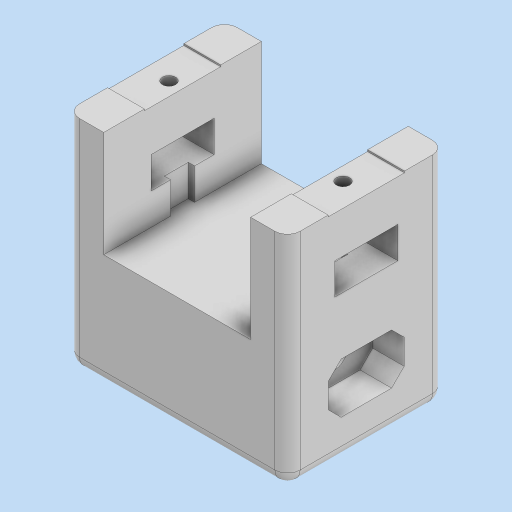
# Autodesk Inventor part: Base_Motor_Hombro2
Saved by Autodesk Inventor 2024 (Build 280153000, 153)
## iProperties
Created: 2024-07-27
Part Number: Base_Motor_Hombro2
Material: Generic
Document SubType Name: Modeling
Designer: MxMon
Density: 1 g/cm^3
Appearance: Default
Author: MxMon
Autodesk Inventor part; units mm, degrees
ref_plane "YZ Plane" through (0, 0, 0) normal (1, 0, 0) x (0, 1, 0)
ref_plane "XZ Plane" through (0, 0, 0) normal (0, 1, 0) x (-1, 0, 0)
sketch "Sketch1" plane through (0, 0, 0) normal (0, 0, 1) x (1, 0, 0)
  line L0 (17.5, 17.4) -> (17.5, -17.4)
  line L1 (17.5, -17.4) -> (-17.5, -17.4)
  line L2 (-17.5, -17.4) -> (-17.5, 17.4)
  line L3 (-17.5, 17.4) -> (17.5, -17.4) construction
  line L4 (17.5, 17.4) -> (-17.5, -17.4) construction
  line L5 (-11.65, 0.6) -> (11.65, 0.6)
  line L6 (-11.65, 0.6) -> (-11.65, 17.4)
  line L7 (11.65, 0.6) -> (11.65, 17.4)
  line L8 (-17.5, 17.4) -> (-11.65, 17.4)
  line L9 (11.65, 17.4) -> (17.5, 17.4)
  line L10 (17.5, -5.4) -> (-17.5, -5.4) construction
  line L11 (17.5, -11.4) -> (-17.5, -11.4) construction
  point P0 (0, 0)
  point P1 (0, 0.6)
  dimension "d0" = 23.3
  dimension "d2" = 6
  dimension "d3" = 16.8
  dimension "d4" = 6
  dimension "d6" = 35
  dimension "d8" = 6
  constraints: 24 end point, 8 perpendicular, 4 point on line, 3 horizontal, 3 midpoint, 3 parallel, 1 vertical alignment
  measures "d0" distance of L5.start L5.end
  measures "d2" distance between parallel lines of L10 L5
  measures "d3" distance of L5.start L6.end
  measures "d4" distance between parallel lines of L11 L10
  measures "d6" distance from line of L0.end L2
  measures "d8" distance between parallel lines of L1 L11
extrude "Extrusion1" add sketch "Sketch1" along normal blind 25
sketch "Sketch2" plane through (-17.5, 17.4, 0) normal (0, 1, 0) x (1, 0, 0)
  line L0 (5.85, 0) -> (5.85, -25) projected
  line L1 (5.85, 0) -> (0, 0) projected
  point P0 (17.5, 0)
  point P1 (3.7, -12.5)
  point P2 (5.85, -12.5)
  dimension "d25" = 2.15
  constraints: 1 horizontal alignment, 1 midpoint
  measures "d25" distance of point (5.85, -12.5) point (3.7, -12.5)
hole "Hole1" at (-13.8, 17.4, 12.5) direction (0, -1, 0) diameter 2.1 depth 8 tip angle 118
sketch "Sketch3" plane through (11.65, 17.4, 0) normal (0, 1, 0) x (1, 0, 0)
  line L0 (0, 0) -> (0, -25) projected
  point P0 (-11.65, 0)
  point P1 (2.15, -12.5)
  point P2 (0, -12.5)
  point P3 (0, -12.5)
  dimension "d27" = 2.15
  constraints: 2 midpoint, 1 horizontal alignment
  measures "d27" distance of point (0, -12.5) point (2.15, -12.5)
hole "Hole2" at (13.8, 17.4, 12.5) direction (0, -1, 0) diameter 2.1 depth 8 tip angle 118
sketch "Sketch4" plane through (17.5, -17.4, 0) normal (1, 0, 0) x (0, 0, -1)
  line L0 (0, 0) -> (-25, 0) projected
  line L1 (0, 34.8) -> (-25, 34.8) projected
  point P0 (0, 17.4)
  point P1 (0, 12)
  point P2 (0, 12)
  point P3 (0, 12)
  point P4 (0, 6)
  point P5 (0, 6)
  point P6 (0, 6)
  point P7 (-12.5, 10)
  point P8 (-12.5, 34.8)
  dimension "d28" = 10
  constraints: 1 midpoint, 1 vertical alignment
  measures "d28" distance from line of point (-12.5, 10) L0
hole "Hole3" at (17.5, -7.4, 12.5) direction (-1, 0, 0) diameter 4 end through all
fillet "Fillet1" radius 2 6 edges at (17.5, 0, 25) (17.5, -17.4, 12.5) (17.5, 0, 0) (-17.5, 0, 0) (-17.5, -17.4, 12.5) (-17.5, 0, 25)
fillet "Fillet2" radius 2 6 edges at (16.9142, -16.8142, 24.4142) (-16.9142, -16.8142, 24.4142) (0, -17.4, 25) (16.9142, -16.8142, 0.5858) (-16.9142, -16.8142, 0.5858) (0, -17.4, 0)
sketch "Sketch5" plane through (11.65, 0.6, 0) normal (-1, 0, 0) x (0, 0, 1)
  line L0 (0, 0) -> (25, 0) projected
  line L1 (17.5, 0) -> (7.5, 0)
  line L2 (7.5, 5) -> (7.5, 10)
  line L3 (7.5, 10) -> (17.5, 10)
  line L4 (17.5, 10) -> (17.5, 5)
  line L5 (7.5, 5) -> (17.5, 5)
  line L6 (0, 16.8) -> (25, 16.8) projected
  point P0 (0, -0.6)
  point P1 (12.5, 0)
  point P2 (12.5, 0)
  point P3 (12.5, 5)
  point P4 (12.5, 16.8)
  point P5 (12.5, 10)
  dimension "d38" = 10
  dimension "d39" = 10
  dimension "d73" = 5
  dimension "d74" = 5
  constraints: 10 end point, 5 midpoint, 2 parallel, 1 coincident, 1 horizontal, 1 perpendicular, 1 point on line, 1 vertical alignment
  measures "d38" distance of L3.end L1.start
  measures "d39" distance of L2.end L3.end
  measures "d73" distance from line of L0 point (12.5, 5)
  measures "d74" distance between parallel lines of L5 L3
extrude "Extrusion2" cut sketch "Sketch5" against normal through all
sketch "Sketch6" plane through (-11.65, 17.4, 25) normal (0, 1, 0) x (1, 0, 0)
  line L0 (-5.85, 2) -> (-5.85, 23) projected
  line L1 (0, 25) -> (0, 0) projected
  line L2 (-5.85, 18.55) -> (0, 18.55)
  line L3 (0, 18.55) -> (0, 6.45)
  line L4 (0, 6.45) -> (-5.85, 6.45)
  line L5 (-5.85, 6.45) -> (-5.85, 18.55)
  point P0 (11.65, 25)
  point P1 (-2.15, 12.5)
  point P2 (-5.85, 12.5)
  point P3 (-5.85, 6.45)
  dimension "d42" = 12.1
  constraints: 8 end point, 2 parallel, 2 point on line, 1 horizontal, 1 horizontal alignment, 1 midpoint, 1 perpendicular
  measures "d42" distance of L4.end L2.start
sketch "Sketch7" plane through (11.65, 17.4, 25) normal (0, 1, 0) x (1, 0, 0)
  line L0 (-11.65, 25) -> (-11.65, 0.0464) construction
  line L1 (-29.15, 18.55) -> (-23.3, 18.55) projected
  line L2 (-29.15, 6.45) -> (-29.15, 18.55) projected
  line L3 (-23.3, 6.45) -> (-29.15, 6.45) projected
  line L4 (-23.3, 18.55) -> (-23.3, 6.45) projected
  line L5 (5.85, 18.55) -> (0, 18.55)
  line L6 (5.85, 6.45) -> (5.85, 18.55)
  line L7 (0, 6.45) -> (5.85, 6.45)
  line L8 (0, 18.55) -> (0, 6.45)
  constraints: 10 end point, 4 symmetric about line, 1 vertical
extrude "Extrusion4" cut sketch "Sketch7" against normal blind 0.25 contours L6 L7 L8 L5
extrude "Extrusion5" cut sketch "Sketch6" against normal blind 0.25
ref_plane "Work Plane1" through (0, -15.4, 2) normal (-1, 0, 0) x (0, 0, 1)
sketch "Sketch10" plane through (0, -15.4, 2) normal (-1, 0, 0) x (0, 0, 1)
  circle A0 centre (10.5, 8) radius 2 projected
  line L0 (10.5, 12.825) -> (6.175, 11.0677)
  line L1 (6.175, 11.0677) -> (6.175, 4.9323)
  line L2 (6.175, 4.9323) -> (10.5, 3.175)
  line L3 (10.5, 3.175) -> (14.825, 4.9323)
  line L4 (14.825, 4.9323) -> (14.825, 11.0677)
  line L5 (14.825, 11.0677) -> (10.5, 12.825)
  line L6 (6.175, 8) -> (14.825, 8)
  arc A1 (8.5, 8) -> (12.5, 8) centre (10.5, 8) ccw
  arc A2 (12.5, 8) -> (8.5, 8) centre (10.5, 8) ccw
  point P0 (-2, 15.4)
  dimension "d50" = 9
  dimension "d52" = 8.65
  dimension "d54" = 9.65
  dimension "d72" = 9
  constraints: 14 end point, 6 point on circle, 3 equal length, 2 centre point, 2 concentric, 2 midpoint, 2 parallel, 2 point on line, 1 horizontal alignment, 1 vertical, 1 vertical alignment
  measures "d50" distance of L0.start L1.end
  measures "d52" distance between parallel lines of L4 L1
  measures "d54" distance of L2.end L0.start
  measures "d72" distance of L0.start L3.end
extrude "Extrusion8" cut sketch "Sketch10" along normal mid plane 3.5 contours A0 L6 L1 L0 L5 L4
sketch "Sketch12" plane through (-15.5, -17.4, 2) normal (0, -1, 0) x (1, 0, 0)
  line L0 (17.25, 12.5) -> (17.25, 8.5) projected
  line L1 (13.75, 8.5) -> (13.75, 12.5) projected
  line L2 (17.25, 14.825) -> (13.75, 14.825) projected
  line L3 (17.25, 6.175) -> (13.75, 6.175)
  line L4 (13.75, 6.175) -> (13.75, 14.825)
  line L5 (13.75, 14.825) -> (17.25, 14.825)
  line L6 (17.25, 14.825) -> (17.25, 6.175)
  line L7 (17.25, 10.5) -> (13.75, 10.5) projected
  line L8 (17.25, 6.175) -> (13.75, 14.825) construction
  line L9 (13.75, 6.175) -> (17.25, 14.825) construction
  point P0 (15.5, -2)
  point P1 (15.5, 10.5)
  constraints: 12 end point, 3 midpoint, 2 parallel, 1 horizontal, 1 perpendicular
extrude "Extrusion9" cut sketch "Sketch12" against normal blind 10.25
sketch "Sketch13" plane through (17.5, -15.4, 23) normal (1, 0, 0) x (0, 0, -1)
  line L0 (4.5, 12) -> (16.5, 12)
  line L1 (16.5, 12) -> (16.5, 4)
  line L2 (16.5, 4) -> (4.5, 4)
  line L3 (4.5, 4) -> (4.5, 12)
  circle A0 centre (10.5, 8) radius 2 projected
  line L4 (4.5, 12) -> (16.5, 4) construction
  line L5 (16.5, 12) -> (4.5, 4) construction
  point P0 (23, 15.4)
  dimension "d65" = 12
  dimension "d66" = 8
  constraints: 12 end point, 2 midpoint, 2 parallel, 1 horizontal, 1 perpendicular
  measures "d65" distance of L1.end L2.end
  measures "d66" distance of L0.end L1.end
extrude "Extrusion10" cut sketch "Sketch13" against normal blind 5
chamfer "Chamfer1" distance 2 angle 45 4 edges at (15, -3.4, 18.5) (15, -3.4, 6.5) (15, -11.4, 6.5) (15, -11.4, 18.5)
sketch "Sketch14" plane through (11.65, 0.6, 0) normal (-1, 0, 0) x (0, 0, 1)
  line L0 (16.7352, 5) -> (8.2648, 5)
  line L1 (14.4, 5) -> (14.4, 0)
  line L2 (0.8122, 0) -> (24.1878, 0)
  line L3 (10.6, 5) -> (10.6, 0)
  line L4 (7.5, 5) -> (17.5, 5) projected
  line L5 (0, 0) -> (25, 0) projected
  point P0 (0, -0.6)
  point P1 (0.8122, 2.1029)
  point P2 (12.5, 0)
  point P3 (11.4122, 7.7029)
  point P4 (11.4122, 2.7029)
  point P5 (6.5, -6)
  point P6 (12.5, 0)
  point P7 (12.5, 5)
  point P8 (10.6, 5)
  point P9 (10.6, 0)
  dimension "d75" = 3.8
  dimension "d76" = 1.9
  constraints: 8 end point, 5 midpoint, 2 horizontal, 2 point on line, 2 vertical, 1 horizontal alignment, 1 parallel
  measures "d75" distance of L1.start L3.start
  measures "d76" distance of point (12.5, 0) L1.end
extrude "Extrusion11" cut sketch "Sketch14" against normal blind 1
mirror "Mirror1" about plane through (0, 0, 0) normal (1, 0, 0) of "Extrusion2", "Extrusion11"
body "Solid1"
